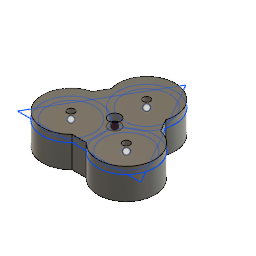
base_bateria (Autodesk Fusion 360 design; units mm, degrees)
Autodesk Fusion 360 part; units mm, degrees
note: some values were not read from the file. Set by a fixed rule: which sketch regions a step uses.
sketch "Sketch1" plane through (0, 0, 0) normal (0, 1, 0) x (1, 0, 0)
  circle A0 centre (0, 13.5) radius 9.75
  circle A1 centre (-11.6913, -6.75) radius 9.75
  circle A2 centre (11.6913, -6.75) radius 9.75
  line L0 (25.9808, -15) -> (0, 30)
  line L1 (0, 30) -> (-25.9808, -15)
  line L2 (-25.9808, -15) -> (25.9808, -15)
  circle A3 centre (0, 13.5) radius 12
  circle A4 centre (-11.6913, -6.75) radius 12
  circle A5 centre (11.6913, -6.75) radius 12
  circle A6 centre (0, 0) radius 2.5
  circle A7 centre (-11.6913, -6.75) radius 1.5
  circle A8 centre (11.6913, -6.75) radius 1.5
  circle A9 centre (0, 13.5) radius 1.5
  dimension "d1" = 19.5
  dimension "d2" = 13.5
  dimension "d4" = 360
  dimension "d5" = 30
  dimension "d6" = 24
  dimension "d8" = 360
  dimension "d9" = 5
  dimension "d14" = 3
  dimension "d16" = 360
  constraint coincident A6.centre origin
  constraint concentric A0 A3
  constraint concentric A4 A7
  measures "d1" diameter of A0
  measures "d2" distance of A6.centre A0.centre
  measures "d5" distance of L0.start A6.centre
  measures "d6" diameter of A3
  measures "d9" diameter of A6
  measures "d14" diameter of A7
extrude "Extrude1" add sketch "Sketch1" along normal blind 3 contours A0 L0 | A0 L0 A3 | A0 L0 L1 | A0 L0 L1 A3 | A0 L0 L1 A3 A4 A5 A6 | A0 L1 | A0 L1 A3 | L0 A3 A5 | L1 A3 A4 | A2 L0 A5 | A2 L0 L2 A3 A4 A5 A6 | A3 A5 | A1 L1 L2 A3 A4 A5 A6 | A1 L1 A4 | A3 A4 | A2 L0 L2 | A2 L0 | A3 A5 A6 | A1 L1 | A1 L1 L2 | A1 L1 L2 A4 | A3 A4 A6 | A2 L2 | A2 L2 A5 | A2 L0 L2 A5 | A1 L2 A4 | L2 A4 A5 | A4 A5 A6 | A1 L2 | A4 A5 | A7 | A8 | A9
extrude "Extrude2" add sketch "Sketch1" against normal blind 10 contours A0 L0 A3 | A0 L0 L1 A3 | A0 L0 L1 A3 A4 A5 A6 | A0 L1 A3 | L0 A3 A5 | L1 A3 A4 | A2 L0 A5 | A2 L0 L2 A3 A4 A5 A6 | A3 A5 | A1 L1 L2 A3 A4 A5 A6 | A1 L1 A4 | A3 A4 | A3 A5 A6 | A1 L1 L2 A4 | A3 A4 A6 | A2 L2 A5 | A2 L0 L2 A5 | A1 L2 A4 | L2 A4 A5 | A4 A5 A6 | A4 A5
extrude "Extrude3" cut sketch "Sketch1" along normal through all contours A7 | A8 | A9
